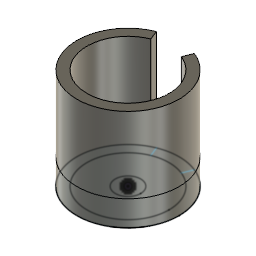
motor_bottom (Autodesk Fusion 360 design; units mm, degrees)
Autodesk Fusion 360 part; units mm, degrees
sketch "スケッチ1" plane through (0, 0, 0) normal (0, 0, 1) x (1, 0, 0)
  circle A0 centre (0, 0) radius 3.25
  circle A1 centre (0, 0) radius 4.05
  circle A2 centre (0, 0) radius 1
  line L0 (-1.5041, 3.7603) -> (-1.207, 3.0175)
  line L1 (1.207, 3.0175) -> (1.5041, 3.7603)
  dimension "d1" = 6.5
  dimension "d2" = 0.8
  dimension "d3" = 2
  constraint coincident A0.centre A1.centre
  constraint coincident A1 L0.start
  constraint coincident A1 L1.end
  constraint coincident A0 L0.end
  constraint coincident A0 L1.start
  measures "d1" diameter of A0
  measures "d3" diameter of A2
extrude "押し出し1" add sketch "スケッチ1" along normal blind 2 makes body 1
extrude "押し出し2" add sketch "スケッチ1" along normal blind 8 separate body contours A0 A1 L0 L1 picked at (3.7683, -0.2009) makes body 2
